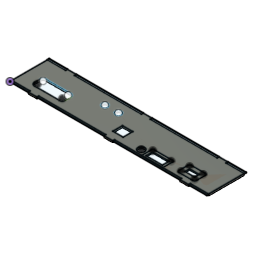
GBS 8200 Rückteil v5 (Autodesk Fusion 360 design; units mm, degrees)
Autodesk Fusion 360 part; units mm, degrees
sketch "Skizze1" plane through (0, 0, 0) normal (0, 1, 0) x (1, 0, 0)
  line L0 (0, 0) -> (204, 0)
  line L1 (204, 0) -> (204, 40.6)
  line L2 (204, 40.6) -> (0, 40.6)
  line L3 (0, 40.6) -> (0, 0)
  line L4 (0, 0) -> (18.8, 0)
  line L5 (18.8, 0) -> (18.8, 1.8)
  line L6 (18.8, 1.8) -> (0, 1.8)
  line L7 (0, 1.8) -> (0, 0)
  line L8 (28, 0) -> (97.4, 0)
  line L9 (97.4, 0) -> (97.4, 1.8)
  line L10 (97.4, 1.8) -> (28, 1.8)
  line L11 (28, 1.8) -> (28, 0)
  line L12 (106.6, 0) -> (176, 0)
  line L13 (176, 0) -> (176, 1.8)
  line L14 (176, 1.8) -> (106.6, 1.8)
  line L15 (106.6, 1.8) -> (106.6, 0)
  line L16 (204, 0) -> (185.2, 0)
  line L17 (185.2, 0) -> (185.2, 1.8)
  line L18 (185.2, 1.8) -> (204, 1.8)
  line L19 (204, 1.8) -> (204, 0)
  line L20 (0, 40.6) -> (18.8, 40.6)
  line L21 (18.8, 40.6) -> (18.8, 38.8)
  line L22 (18.8, 38.8) -> (0, 38.8)
  line L23 (0, 38.8) -> (0, 40.6)
  line L24 (97.4, 40.6) -> (28, 40.6)
  line L25 (28, 40.6) -> (28, 38.8)
  line L26 (28, 38.8) -> (97.4, 38.8)
  line L27 (97.4, 38.8) -> (97.4, 40.6)
  line L28 (204, 40.6) -> (185.2, 40.6)
  line L29 (185.2, 40.6) -> (185.2, 38.8)
  line L30 (185.2, 38.8) -> (204, 38.8)
  line L31 (204, 38.8) -> (204, 40.6)
  line L32 (176, 40.6) -> (106.6, 40.6)
  line L33 (106.6, 40.6) -> (106.6, 38.8)
  line L34 (106.6, 38.8) -> (176, 38.8)
  line L35 (176, 38.8) -> (176, 40.6)
  line L36 (42.59, 20.6) -> (16.59, 20.6)
  line L37 (13.59, 17.6) -> (13.59, 11.6)
  line L38 (16.59, 8.6) -> (42.59, 8.6)
  line L39 (45.59, 11.6) -> (45.59, 17.6)
  arc A0 (16.59, 20.6) -> (13.59, 17.6) centre (16.59, 17.6) ccw
  arc A1 (13.59, 11.6) -> (16.59, 8.6) centre (16.59, 11.6) ccw
  arc A2 (45.59, 17.6) -> (42.59, 20.6) centre (42.59, 17.6) ccw
  arc A3 (42.59, 8.6) -> (45.59, 11.6) centre (42.59, 11.6) ccw
  line L40 (97.99, 18.6) -> (108.69, 18.6)
  line L41 (108.69, 18.6) -> (108.69, 8.6)
  line L42 (108.69, 8.6) -> (97.99, 8.6)
  line L43 (97.99, 8.6) -> (97.99, 18.6)
  circle A4 centre (129.19, 6.9) radius 3.5
  line L44 (137.19, 10.8) -> (154.09, 10.8)
  line L45 (154.09, 10.8) -> (154.09, 3.8)
  line L46 (154.09, 3.8) -> (137.19, 3.8)
  line L47 (137.19, 3.8) -> (137.19, 10.8)
  line L48 (171.59, 14.6) -> (181.59, 14.6)
  line L49 (181.59, 14.6) -> (181.59, 9.8)
  line L50 (181.59, 9.8) -> (171.59, 9.8)
  line L51 (171.59, 9.8) -> (171.59, 14.6)
  circle A5 centre (70.59, 27.8) radius 3
  circle A6 centre (84.59, 27.8) radius 3
  line L52 (169.59, 18.6) -> (183.59, 18.6)
  line L53 (185.59, 16.6) -> (185.59, 7.8)
  line L54 (183.59, 5.8) -> (169.59, 5.8)
  line L55 (167.59, 7.8) -> (167.59, 16.6)
  arc A7 (169.59, 18.6) -> (167.59, 16.6) centre (169.59, 16.6) ccw
  arc A8 (185.59, 16.6) -> (183.59, 18.6) centre (183.59, 16.6) ccw
  arc A9 (167.59, 7.8) -> (169.59, 5.8) centre (169.59, 7.8) ccw
  arc A10 (183.59, 5.8) -> (185.59, 7.8) centre (183.59, 7.8) ccw
  line L56 (134.69, 1.8) -> (156.59, 1.8)
  line L57 (156.59, 1.8) -> (156.59, 11.8)
  line L58 (155.09, 13.3) -> (136.19, 13.3)
  line L59 (134.69, 11.8) -> (134.69, 1.8)
  arc A11 (136.19, 13.3) -> (134.69, 11.8) centre (136.19, 11.8) ccw
  arc A12 (156.59, 11.8) -> (155.09, 13.3) centre (155.09, 11.8) ccw
  dimension "d1" = 204
  dimension "d2" = 40.6
  dimension "d3" = 18.8
  dimension "d4" = 1.8
  dimension "d6" = 1.8
  dimension "d7" = 9.2
  dimension "d8" = 97.4
  dimension "d10" = 1.8
  dimension "d11" = 9.2
  dimension "d12" = 18.8
  dimension "d13" = 1.8
  dimension "d14" = 9.2
  dimension "d15" = 18.8
  dimension "d16" = 1.8
  dimension "d18" = 1.8
  dimension "d19" = 9.2
  dimension "d20" = 97.4
  dimension "d21" = 18.8
  dimension "d22" = 1.8
  dimension "d24" = 1.8
  dimension "d25" = 9.2
  dimension "d26" = 9.2
  dimension "d39" = 6.8
  dimension "d40" = 3
  dimension "d41" = 3
  dimension "d42" = 3
  dimension "d43" = 3
  dimension "d91" = 13.59
  dimension "d92" = 52.4
  dimension "d93" = 6.8
  dimension "d94" = 10.7
  dimension "d95" = 10
  dimension "d96" = 7
  dimension "d97" = 20.5
  dimension "d98" = 5.1
  dimension "d99" = 8
  dimension "d100" = 16.9
  dimension "d101" = 2
  dimension "d102" = 7
  dimension "d103" = 17.5
  dimension "d104" = 10
  dimension "d105" = 8
  dimension "d106" = 4.8
  dimension "d110" = 14
  dimension "d114" = 11
  dimension "d115" = 11
  dimension "d116" = 6
  dimension "d117" = 6
  dimension "d118" = 4
  dimension "d119" = 4
  dimension "d120" = 4
  dimension "d121" = 4
  dimension "d122" = 2
  dimension "d123" = 2
  dimension "d124" = 2
  dimension "d125" = 2
  dimension "d126" = 2.5
  dimension "d127" = 2.5
  dimension "d128" = 2.5
  dimension "d143" = 1.5
  dimension "d144" = 1.5
  constraint horizontal L0
  constraint vertical L1
  constraint horizontal L2
  constraint vertical L3
  constraint coincident L0.start L3.end
  constraint horizontal L4
  constraint vertical L5
  constraint horizontal L6
  constraint vertical L7
  constraint horizontal L8
  constraint vertical L9
  constraint horizontal L10
  constraint vertical L11
  constraint coincident L0 L8.start
  constraint horizontal L12
  constraint vertical L13
  constraint horizontal L14
  constraint vertical L15
  constraint coincident L0 L12.start
  constraint horizontal L16
  constraint vertical L17
  constraint horizontal L18
  constraint vertical L19
  constraint horizontal L20
  constraint vertical L21
  constraint horizontal L22
  constraint vertical L23
  constraint horizontal L24
  constraint vertical L25
  constraint horizontal L26
  constraint vertical L27
  constraint coincident L2 L24.start
  constraint horizontal L28
  constraint vertical L29
  constraint horizontal L30
  constraint vertical L31
  constraint horizontal L32
  constraint vertical L33
  constraint horizontal L34
  constraint vertical L35
  constraint coincident L2 L32.start
  constraint horizontal L36
  constraint vertical L37
  constraint horizontal L38
  constraint vertical L39
  constraint tangent L37 A0
  constraint tangent L36 A0
  constraint tangent L37 A1
  constraint tangent L38 A1
  constraint tangent L36 A2
  constraint tangent L39 A2
  constraint tangent L39 A3
  constraint tangent L38 A3
  constraint horizontal L40
  constraint vertical L41
  constraint horizontal L42
  constraint vertical L43
  constraint horizontal L44
  constraint vertical L45
  constraint horizontal L46
  constraint vertical L47
  constraint horizontal L48
  constraint vertical L49
  constraint horizontal L50
  constraint vertical L51
  constraint horizontal L52
  constraint vertical L53
  constraint horizontal L54
  constraint vertical L55
  constraint tangent L52 A7
  constraint tangent L55 A7
  constraint tangent L52 A8
  constraint tangent L53 A8
  constraint tangent L55 A9
  constraint tangent L54 A9
  constraint tangent L53 A10
  constraint tangent L54 A10
  constraint horizontal L56
  constraint vertical L57
  constraint horizontal L58
  constraint vertical L59
  constraint coincident L14 L56.start
  constraint tangent L58 A11
  constraint tangent L59 A11
  constraint tangent L58 A12
  constraint tangent L57 A12
  measures "d1" distance of L0.start L0.end
  measures "d2" distance of L0.start L2.end
  measures "d3" distance of L0.start L4.end
  measures "d4" distance of L0.start L6.end
  measures "d6" distance of L8.start L10.end
  measures "d7" distance of L4.end L8.start
  measures "d8" distance of L3 L9
  measures "d10" distance of L12.start L14.end
  measures "d11" distance of L8.end L12.start
  measures "d12" distance of L0.end L16.end
  measures "d13" distance of L0.end L18.end
  measures "d14" distance of L13.end L17.end
  measures "d15" distance of L2.end L20.end
  measures "d16" distance of L2.end L22.end
  measures "d18" distance of L24.start L26.end
  measures "d19" distance of L21.end L25.end
  measures "d20" distance of L22.end L26.end
  measures "d21" distance of L1.end L28.end
  measures "d22" distance of L1.end L30.end
  measures "d24" distance of L32.start L34.end
  measures "d25" distance of L28.end L32.start
  measures "d26" distance of L26.end L33.end
  measures "d39" distance of L10 L38
  measures "d40" radius of A0
  measures "d41" radius of A1
  measures "d42" radius of A2
  measures "d43" radius of A3
  measures "d91" distance of L3 L37
  measures "d92" distance of L39 L43
  measures "d93" distance of L14 L42
  measures "d94" distance of L40.start L40.end
  measures "d95" distance of L40 L42
  measures "d96" diameter of A4
  measures "d97" distance of L41 A4.centre
  measures "d98" distance of L14 A4.centre
  measures "d99" distance of A4.centre L47
  measures "d100" distance of L44.start L44.end
  measures "d101" distance of L14 L46
  measures "d102" distance of L44.end L46
  measures "d103" distance of L45 L51
  measures "d104" distance of L48.start L48.end
  measures "d105" distance of L14 L50.end
  measures "d106" distance of L48.end L49.end
  measures "d110" horizontal distance of A5.centre A6.centre
  measures "d114" distance of L26 A5.centre
  measures "d115" distance of L26 A6.centre
  measures "d116" diameter of A5
  measures "d117" diameter of A6
  measures "d118" distance of L51 L55
  measures "d119" distance of L49 L53
  measures "d120" distance of L48 L52
  measures "d121" distance of L50 L54
  measures "d122" radius of A7
  measures "d123" radius of A8
  measures "d124" radius of A9
  measures "d125" radius of A10
  measures "d126" distance of L47 L59
  measures "d127" distance of L45 L57
  measures "d128" distance of L44 L58
  measures "d143" radius of A11
  measures "d144" radius of A12
extrude "Extrusion22" add sketch "Skizze1" against normal blind 1.8 contours L0 L1 L2 L3 L5 L6 L9 L10 L11 L13 L14 L15 L17 L18 L21 L22 L25 L26 L27 L29 L30 L33 L34 L35 L57 L58 L59 A11 A12
extrude "Extrusion23" add sketch "Skizze1" against normal blind 1.2 contours L14 L56 L57 L58 L59 A11 A12 | L52 L53 L54 L55 A7 A8 A9 A10
extrude "Extrusion1" [suppressed]
extrude "Extrusion2" [suppressed]
extrude "Extrusion3" [suppressed]
extrude "Extrusion4" [suppressed]
extrude "Extrusion5" [suppressed]
